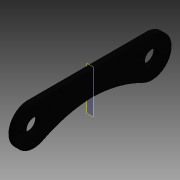
# Autodesk Inventor part: tibia extrude
Saved by Autodesk Inventor 2015 (Build 190159000, 159)
## iProperties
Created: 2015-01-13
Part Number: tibia extrude
Material: Generic
Document SubType Name: Modeling
Designer: I Was ME
Density: 1 g/cm^3
Appearance: Anodized - Black
Mass: 6.09817 g
Surface Area: 48.2309 cm^2
Volume: 6.09817 cm^3
Author: I Was ME
Autodesk Inventor part; units mm, degrees
ref_plane "YZ Plane" through (0, 0, 0) normal (1, 0, 0) x (0, 1, 0)
ref_plane "XZ Plane" through (0, 0, 0) normal (0, 1, 0) x (-1, 0, 0)
ref_plane "XY Plane" through (0, 0, 0) normal (0, 0, 1) x (1, 0, 0)
sketch "Sketch1" plane through (0, 0, 0) normal (1, 0, 0) x (0, 1, 0)
  line L0 (0, 24.9554) -> (36.4449, 24.9554)
  arc A0 (31.5833, 1.489) -> (36.4449, 24.9554) centre (37.5, 12.5) ccw
  arc A1 (31.7956, 1.3803) -> (0, 9.582) centre (-2.2398, -64.8326) ccw
  circle A2 centre (37.5, 3.991) radius 1.25
  circle A3 centre (28.991, 12.5) radius 1.25
  circle A4 centre (37.5, 21.009) radius 1.25
  circle A5 centre (46.009, 12.5) radius 1.25
  circle A6 centre (28.6546, 17.1646) radius 1.25
  circle A7 centre (20.6937, 21.3627) radius 1.25
  circle A8 centre (37.5, 12.5) radius 4.5
  line L1 (-2.2398, 24.9554) -> (-2.25, 24.9554)
  arc A9 (-2.2398, 9.6157) -> (-2.25, 9.6157) centre (-2.2398, -64.8326) ccw
  arc A10 (0, 9.582) -> (-31.7956, 1.3803) centre (2.2398, -64.8326) ccw
  line L2 (0, 24.9554) -> (-36.4449, 24.9554)
  arc A11 (-36.4449, 24.9554) -> (-31.5833, 1.489) centre (-37.5, 12.5) ccw
  circle A12 centre (-37.5, 3.991) radius 1.25
  circle A13 centre (-28.991, 12.5) radius 1.25
  circle A14 centre (-37.5, 21.009) radius 1.25
  circle A15 centre (-46.009, 12.5) radius 1.25
  circle A16 centre (-28.6546, 17.1646) radius 1.25
  circle A17 centre (-20.6937, 21.3627) radius 1.25
  circle A18 centre (-37.5, 12.5) radius 4.5
  line L3 (2.2398, 24.9554) -> (2.25, 24.9554)
  arc A19 (2.25, 9.6157) -> (2.2398, 9.6157) centre (2.2398, -64.8326) ccw
  point P0 (0.0204, 0)
  point P1 (-0.0204, 0)
  dimension "d47" = 8.509
  dimension "d48" = 8.509
  dimension "d49" = 8.509
  dimension "d50" = 8.509
  dimension "d51" = 10
  dimension "d53" = 9
  dimension "d56" = 9
  dimension "d58" = 4.1981
  dimension "d61" = 75
  constraints: 20 centre point, 14 point on circle, 8 end point, 4 horizontal alignment, 2 coincident, 2 vertical alignment, 1 horizontal
  measures "d47" distance of A2.centre A0.centre
  measures "d48" distance of A4.centre A0.centre
  measures "d49" distance of A5.centre A0.centre
  measures "d50" distance of A3.centre A0.centre
  measures "d51" distance of A6.centre A0.centre
  measures "d53" distance of A6.centre A7.centre
  measures "d56" diameter of A8
  measures "d58" vertical distance of A7.centre A6.centre
  measures "d61" distance of A0.centre A11.centre
extrude "Extrusion3" add sketch "Sketch1" along normal mid plane 3.5
body "Solid3"
